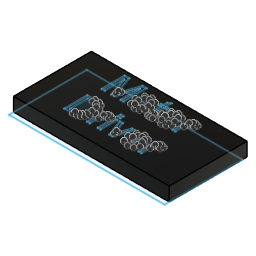
Motor Driver (Autodesk Fusion 360 design; units mm, degrees)
Autodesk Fusion 360 part; units mm, degrees
sketch "sketch 914" plane through (0, 0, 41) normal (0, 0, 1) x (1, 0, 0)
  line L0 (19, -12) -> (-15, -12)
  line L1 (19, 5) -> (19, -12)
  line L2 (-15, 5) -> (19, 5)
  line L3 (-15, -12) -> (-15, 5)
extrude "Extrude1" add sketch "sketch 914" along normal blind 3
sketch "sketch 936" plane through (0, 0, 44) normal (0, 0, 1) x (-1, 0, 0)
  spline S0 degree 3 poles (-7.3462, 7.2033) (-7.4233, 7.1305) (-7.5921, 6.9711) (-7.6781, 6.7547) (-7.7248, 6.6371) knots 0 0 0 0 0.031433 0.068842 0.068842 0.068842 0.068842
  spline S1 degree 3 poles (-6.7698, 7.3806) (-6.8767, 7.3743) (-7.0836, 7.3621) (-7.2607, 7.255) (-7.3462, 7.2033) knots 0 0 0 0 0.031605 0.061119 0.061119 0.061119 0.061119
  spline S2 degree 3 poles (-6.0126, 7.0634) (-6.1207, 7.1559) (-6.339, 7.3427) (-6.6253, 7.3679) (-6.7698, 7.3806) knots 0 0 0 0 0.041584 0.083942 0.083942 0.083942 0.083942
  spline S3 degree 3 poles (-5.675, 6.1494) (-5.6927, 6.3313) (-5.7254, 6.6668) (-5.9224, 6.9388) (-6.0126, 7.0634) knots 0 0 0 0 0.053662 0.09901 0.09901 0.09901 0.09901
  line L0 (-8.3762, 6.1494) -> (-5.675, 6.1494)
  spline S4 degree 3 poles (-8.3796, 5.9857) (-8.3794, 6.0084) (-8.3789, 6.063) (-8.3772, 6.1176) (-8.3762, 6.1494) knots 0 0 0 0 0.006822 0.016375 0.016375 0.016375 0.016375
  spline S5 degree 3 poles (-7.9192, 4.5941) (-8.0532, 4.7859) (-8.3441, 5.202) (-8.3672, 5.7112) (-8.3796, 5.9857) knots 0 0 0 0 0.068809 0.149275 0.149275 0.149275 0.149275
  spline S6 degree 3 poles (-6.7323, 4.0996) (-6.9617, 4.1184) (-7.4113, 4.1554) (-7.7522, 4.4499) (-7.9192, 4.5941) knots 0 0 0 0 0.067144 0.131583 0.131583 0.131583 0.131583
  spline S7 degree 3 poles (-5.5113, 4.6044) (-5.6826, 4.4572) (-6.0337, 4.1556) (-6.4958, 4.1186) (-6.7323, 4.0996) knots 0 0 0 0 0.065997 0.1352 0.1352 0.1352 0.1352
  spline S8 degree 3 poles (-5.0406, 6.0232) (-5.0534, 5.7434) (-5.0771, 5.224) (-5.3742, 4.8) (-5.5113, 4.6044) knots 0 0 0 0 0.082022 0.152248 0.152248 0.152248 0.152248
  spline S9 degree 3 poles (-5.5061, 7.396) (-5.3706, 7.2068) (-5.0776, 6.7982) (-5.0535, 6.294) (-5.0406, 6.0232) knots 0 0 0 0 0.068378 0.147724 0.147724 0.147724 0.147724
  spline S10 degree 3 poles (-6.7664, 7.8854) (-6.5192, 7.869) (-6.0464, 7.8377) (-5.6806, 7.5386) (-5.5061, 7.396) knots 0 0 0 0 0.072283 0.138227 0.138227 0.138227 0.138227
  spline S11 degree 3 poles (-7.8032, 7.5784) (-7.6531, 7.6679) (-7.3343, 7.8578) (-6.9628, 7.8758) (-6.7664, 7.8854) knots 0 0 0 0 0.051631 0.10961 0.10961 0.10961 0.10961
  spline S12 degree 3 poles (-8.3591, 6.7156) (-8.3009, 6.8886) (-8.1881, 7.2236) (-7.9286, 7.4628) (-7.8032, 7.5784) knots 0 0 0 0 0.053808 0.104129 0.104129 0.104129 0.104129
  line L1 (-7.7248, 6.6371) -> (-8.3591, 6.7156)
  spline S13 degree 3 poles (-6.028, 4.8874) (-5.9425, 4.993) (-5.7635, 5.2141) (-5.7277, 5.4969) (-5.7091, 5.6446) knots 0 0 0 0 0.039943 0.083623 0.083623 0.083623 0.083623
  spline S14 degree 3 poles (-6.7391, 4.6044) (-6.6044, 4.6155) (-6.3383, 4.6376) (-6.1305, 4.8049) (-6.028, 4.8874) knots 0 0 0 0 0.039562 0.078122 0.078122 0.078122 0.078122
  spline S15 degree 3 poles (-7.4997, 4.9591) (-7.3943, 4.8556) (-7.1827, 4.6478) (-6.8874, 4.6189) (-6.7391, 4.6044) knots 0 0 0 0 0.042919 0.086214 0.086214 0.086214 0.086214
  spline S16 degree 3 poles (-7.7316, 5.6446) (-7.7161, 5.5075) (-7.6882, 5.2613) (-7.5575, 5.0519) (-7.4997, 4.9591) knots 0 0 0 0 0.040752 0.073178 0.073178 0.073178 0.073178
  line L2 (-5.7091, 5.6446) -> (-7.7316, 5.6446)
  line L3 (-3.3319, 7.8035) -> (-2.7589, 7.8035)
  line L4 (-4.7029, 4.1814) -> (-3.3319, 7.8035)
  line L5 (-4.072, 4.1814) -> (-4.7029, 4.1814)
  line L6 (-3.2671, 6.3915) -> (-4.072, 4.1814)
  spline S17 degree 3 poles (-3.0385, 7.0805) (-3.0704, 6.9751) (-3.1404, 6.7434) (-3.2224, 6.5156) (-3.2671, 6.3915) knots 0 0 0 0 0.033037 0.072597 0.072597 0.072597 0.072597
  spline S18 degree 3 poles (-2.8066, 6.3506) (-2.848, 6.4696) (-2.932, 6.7108) (-3.0027, 6.9562) (-3.0385, 7.0805) knots 0 0 0 0 0.037803 0.076597 0.076597 0.076597 0.076597
  line L7 (-2.029, 4.1814) -> (-2.8066, 6.3506)
  line L8 (-1.381, 4.1814) -> (-2.029, 4.1814)
  line L9 (-2.7589, 7.8035) -> (-1.381, 4.1814)
  line L10 (-0.8182, 7.8035) -> (-0.2043, 7.8035)
  line L11 (-0.8182, 4.1814) -> (-0.8182, 7.8035)
  line L12 (-0.2043, 4.1814) -> (-0.8182, 4.1814)
  line L13 (-0.2043, 7.8035) -> (-0.2043, 4.1814)
  line L14 (-0.8182, 3.5095) -> (-0.2043, 3.5095)
  line L15 (-0.8182, 2.8035) -> (-0.8182, 3.5095)
  line L16 (-0.2043, 2.8035) -> (-0.8182, 2.8035)
  line L17 (-0.2043, 3.5095) -> (-0.2043, 2.8035)
  line L18 (1.5181, 7.8035) -> (2.132, 7.8035)
  line L19 (1.5181, 5.9072) -> (1.5181, 7.8035)
  spline S19 degree 3 poles (1.4158, 5.191) (1.4456, 5.3046) (1.5072, 5.5394) (1.5144, 5.782) (1.5181, 5.9072) knots 0 0 0 0 0.035125 0.072559 0.072559 0.072559 0.072559
  spline S20 degree 3 poles (1.1872, 4.855) (1.2372, 4.9004) (1.3402, 4.9939) (1.3901, 5.124) (1.4158, 5.191) knots 0 0 0 0 0.019933 0.041138 0.041138 0.041138 0.041138
  spline S21 degree 3 poles (0.8257, 4.734) (0.8911, 4.739) (1.0217, 4.7491) (1.1321, 4.8197) (1.1872, 4.855) knots 0 0 0 0 0.019338 0.038658 0.038658 0.038658 0.038658
  spline S22 degree 3 poles (0.3755, 4.867) (0.4489, 4.8282) (0.5902, 4.7536) (0.7493, 4.7403) (0.8257, 4.734) knots 0 0 0 0 0.024622 0.047376 0.047376 0.047376 0.047376
  line L20 (0.1641, 4.2974) -> (0.3755, 4.867)
  spline S23 degree 3 poles (0.795, 4.0996) (0.6887, 4.1094) (0.4645, 4.1301) (0.2676, 4.2398) (0.1641, 4.2974) knots 0 0 0 0 0.031681 0.066776 0.066776 0.066776 0.066776
  spline S24 degree 3 poles (1.189, 4.2224) (1.1279, 4.1866) (1.0061, 4.1151) (0.8652, 4.1048) (0.795, 4.0996) knots 0 0 0 0 0.020935 0.041755 0.041755 0.041755 0.041755
  spline S25 degree 3 poles (1.5795, 4.7306) (1.5179, 4.619) (1.4132, 4.4292) (1.2544, 4.2827) (1.189, 4.2224) knots 0 0 0 0 0.037894 0.064453 0.064453 0.064453 0.064453
  line L21 (1.5795, 4.1814) -> (1.5795, 4.7306)
  line L22 (2.132, 4.1814) -> (1.5795, 4.1814)
  line L23 (2.132, 7.8035) -> (2.132, 4.1814)
  line L24 (-9.737, 7.8035) -> (-9.1231, 7.8035)
  line L25 (-9.737, 5.9072) -> (-9.737, 7.8035)
  spline S26 degree 3 poles (-9.8394, 5.191) (-9.8095, 5.3046) (-9.7479, 5.5394) (-9.7407, 5.782) (-9.737, 5.9072) knots 0 0 0 0 0.035125 0.072559 0.072559 0.072559 0.072559
  spline S27 degree 3 poles (-10.0679, 4.855) (-10.018, 4.9004) (-9.9149, 4.9939) (-9.8651, 5.124) (-9.8394, 5.191) knots 0 0 0 0 0.019933 0.041138 0.041138 0.041138 0.041138
  spline S28 degree 3 poles (-10.4294, 4.734) (-10.364, 4.739) (-10.2334, 4.7491) (-10.123, 4.8197) (-10.0679, 4.855) knots 0 0 0 0 0.019338 0.038658 0.038658 0.038658 0.038658
  spline S29 degree 3 poles (-10.8796, 4.867) (-10.8062, 4.8282) (-10.6649, 4.7536) (-10.5058, 4.7403) (-10.4294, 4.734) knots 0 0 0 0 0.024622 0.047376 0.047376 0.047376 0.047376
  line L26 (-11.0911, 4.2974) -> (-10.8796, 4.867)
  spline S30 degree 3 poles (-10.4601, 4.0996) (-10.5664, 4.1094) (-10.7906, 4.1301) (-10.9876, 4.2398) (-11.0911, 4.2974) knots 0 0 0 0 0.031681 0.066775 0.066775 0.066775 0.066775
  spline S31 degree 3 poles (-10.0662, 4.2224) (-10.1272, 4.1866) (-10.2491, 4.1151) (-10.3899, 4.1048) (-10.4601, 4.0996) knots 0 0 0 0 0.020935 0.041755 0.041755 0.041755 0.041755
  spline S32 degree 3 poles (-9.6756, 4.7306) (-9.7372, 4.619) (-9.8419, 4.4292) (-10.0007, 4.2827) (-10.0662, 4.2224) knots 0 0 0 0 0.037894 0.064453 0.064453 0.064453 0.064453
  line L27 (-9.6756, 4.1814) -> (-9.6756, 4.7306)
  line L28 (-9.1231, 4.1814) -> (-9.6756, 4.1814)
  line L29 (-9.1231, 7.8035) -> (-9.1231, 4.1814)
  line L30 (5.2868, 7.8035) -> (7.0911, 7.8035)
  spline S33 degree 3 poles (4.4836, 7.7183) (4.6084, 7.7431) (4.8735, 7.7959) (5.1438, 7.8009) (5.2868, 7.8035) knots 0 0 0 0 0.0381 0.080914 0.080914 0.080914 0.080914
  spline S34 degree 3 poles (3.8868, 7.4676) (3.976, 7.52) (4.1637, 7.6302) (4.3736, 7.688) (4.4836, 7.7183) knots 0 0 0 0 0.030916 0.064986 0.064986 0.064986 0.064986
  spline S35 degree 3 poles (3.4314, 7.014) (3.5004, 7.1035) (3.6323, 7.2749) (3.8045, 7.4053) (3.8868, 7.4676) knots 0 0 0 0 0.03373 0.064527 0.064527 0.064527 0.064527
  spline S36 degree 3 poles (3.0904, 6.2858) (3.1353, 6.4225) (3.2196, 6.6792) (3.364, 6.9073) (3.4314, 7.014) knots 0 0 0 0 0.042972 0.080682 0.080682 0.080682 0.080682
  spline S37 degree 3 poles (2.9574, 5.2763) (2.9616, 5.4563) (2.9696, 5.7977) (3.0516, 6.1291) (3.0904, 6.2858) knots 0 0 0 0 0.05382 0.1021 0.1021 0.1021 0.1021
  spline S38 degree 3 poles (3.1535, 4.0877) (3.0963, 4.272) (2.9763, 4.659) (2.9639, 5.0641) (2.9574, 5.2763) knots 0 0 0 0 0.05763 0.12096 0.12096 0.12096 0.12096
  spline S39 degree 3 poles (3.7452, 3.2333) (3.6211, 3.354) (3.3681, 3.6) (3.2259, 3.9231) (3.1535, 4.0877) knots 0 0 0 0 0.051428 0.1048 0.1048 0.1048 0.1048
  spline S40 degree 3 poles (4.4785, 2.8752) (4.3419, 2.9136) (4.0756, 2.9886) (3.8534, 3.1532) (3.7452, 3.2333) knots 0 0 0 0 0.042175 0.082214 0.082214 0.082214 0.082214
  spline S41 degree 3 poles (5.3687, 2.8035) (5.1968, 2.8043) (4.8981, 2.8055) (4.6036, 2.8544) (4.4785, 2.8752) knots 0 0 0 0 0.051447 0.089431 0.089431 0.089431 0.089431
  line L31 (7.0911, 2.8035) -> (5.3687, 2.8035)
  line L32 (7.0911, 7.8035) -> (7.0911, 2.8035)
  line L33 (6.4294, 3.3936) -> (6.4294, 7.2135)
  line L34 (5.3789, 3.3936) -> (6.4294, 3.3936)
  spline S42 degree 3 poles (4.5229, 3.4959) (4.638, 3.4663) (4.9182, 3.3942) (5.2081, 3.3938) (5.3789, 3.3936) knots 0 0 0 0 0.035542 0.08651 0.08651 0.08651 0.08651
  spline S43 degree 3 poles (3.897, 4.0604) (3.9833, 3.9332) (4.1463, 3.6934) (4.4024, 3.559) (4.5229, 3.4959) knots 0 0 0 0 0.045283 0.085444 0.085444 0.085444 0.085444
  spline S44 degree 3 poles (3.6395, 5.266) (3.644, 5.0309) (3.6521, 4.6111) (3.8222, 4.2286) (3.897, 4.0604) knots 0 0 0 0 0.069662 0.124385 0.124385 0.124385 0.124385
  spline S45 degree 3 poles (3.7708, 6.2295) (3.7326, 6.0838) (3.6498, 5.7682) (3.6431, 5.4417) (3.6395, 5.266) knots 0 0 0 0 0.045044 0.097543 0.097543 0.097543 0.097543
  spline S46 degree 3 poles (4.1374, 6.8622) (4.0622, 6.7735) (3.9022, 6.5848) (3.8163, 6.3526) (3.7708, 6.2295) knots 0 0 0 0 0.034627 0.073625 0.073625 0.073625 0.073625
  spline S47 degree 3 poles (4.5859, 7.1214) (4.4988, 7.0894) (4.3341, 7.0289) (4.2004, 6.9156) (4.1374, 6.8622) knots 0 0 0 0 0.027605 0.052162 0.052162 0.052162 0.052162
  spline S48 degree 3 poles (5.3619, 7.2135) (5.214, 7.2121) (4.9517, 7.2095) (4.697, 7.1482) (4.5859, 7.1214) knots 0 0 0 0 0.044185 0.078357 0.078357 0.078357 0.078357
  line L35 (6.4294, 7.2135) -> (5.3619, 7.2135)
  line L36 (-9.3516, 0) -> (-8.7377, 0)
  line L37 (-9.3516, -1.8963) -> (-9.3516, 0)
  spline S49 degree 3 poles (-9.454, -2.6126) (-9.4241, -2.4989) (-9.3625, -2.2642) (-9.3553, -2.0215) (-9.3516, -1.8963) knots 0 0 0 0 0.035125 0.07256 0.07256 0.07256 0.07256
  spline S50 degree 3 poles (-9.6825, -2.9485) (-9.6325, -2.9032) (-9.5295, -2.8097) (-9.4797, -2.6796) (-9.454, -2.6126) knots 0 0 0 0 0.019933 0.041138 0.041138 0.041138 0.041138
  spline S51 degree 3 poles (-10.044, -3.0696) (-9.9786, -3.0645) (-9.848, -3.0545) (-9.7376, -2.9838) (-9.6825, -2.9485) knots 0 0 0 0 0.019338 0.038658 0.038658 0.038658 0.038658
  spline S52 degree 3 poles (-10.4942, -2.9366) (-10.4208, -2.9753) (-10.2795, -3.05) (-10.1204, -3.0632) (-10.044, -3.0696) knots 0 0 0 0 0.024622 0.047376 0.047376 0.047376 0.047376
  line L38 (-10.7057, -3.5061) -> (-10.4942, -2.9366)
  spline S53 degree 3 poles (-10.0747, -3.704) (-10.181, -3.6942) (-10.4052, -3.6735) (-10.6022, -3.5638) (-10.7057, -3.5061) knots 0 0 0 0 0.031681 0.066775 0.066775 0.066775 0.066775
  spline S54 degree 3 poles (-9.6808, -3.5812) (-9.7418, -3.617) (-9.8637, -3.6884) (-10.0045, -3.6988) (-10.0747, -3.704) knots 0 0 0 0 0.020935 0.041755 0.041755 0.041755 0.041755
  spline S55 degree 3 poles (-9.2902, -3.073) (-9.3518, -3.1846) (-9.4565, -3.3743) (-9.6153, -3.5208) (-9.6808, -3.5812) knots 0 0 0 0 0.037894 0.064453 0.064453 0.064453 0.064453
  line L39 (-9.2902, -3.6221) -> (-9.2902, -3.073)
  line L40 (-8.7377, -3.6221) -> (-9.2902, -3.6221)
  line L41 (-8.7377, 0) -> (-8.7377, -3.6221)
  spline S56 degree 3 poles (-5.1003, -0.4059) (-4.9637, -0.5975) (-4.6656, -1.0159) (-4.6434, -1.5315) (-4.6313, -1.8111) knots 0 0 0 0 0.069132 0.150979 0.150979 0.150979 0.150979
  spline S57 degree 3 poles (-6.3298, 0.0819) (-6.0912, 0.0644) (-5.6293, 0.0305) (-5.2727, -0.2637) (-5.1003, -0.4059) knots 0 0 0 0 0.06984 0.135217 0.135217 0.135217 0.135217
  spline S58 degree 3 poles (-7.2046, -0.1398) (-7.0673, -0.0752) (-6.7901, 0.0553) (-6.4842, 0.073) (-6.3298, 0.0819) knots 0 0 0 0 0.045086 0.090997 0.090997 0.090997 0.090997
  spline S59 degree 3 poles (-7.8151, -0.7623) (-7.737, -0.636) (-7.5803, -0.3827) (-7.3301, -0.221) (-7.2046, -0.1398) knots 0 0 0 0 0.043936 0.088163 0.088163 0.088163 0.088163
  spline S60 degree 3 poles (-8.0249, -1.8622) (-8.0208, -1.6513) (-8.0134, -1.2718) (-7.8761, -0.919) (-7.8151, -0.7623) knots 0 0 0 0 0.062677 0.112748 0.112748 0.112748 0.112748
  spline S61 degree 3 poles (-7.5508, -3.2145) (-7.6889, -3.0274) (-7.9846, -2.6269) (-8.0109, -2.128) (-8.0249, -1.8622) knots 0 0 0 0 0.068269 0.146129 0.146129 0.146129 0.146129
  spline S62 degree 3 poles (-6.3298, -3.704) (-6.5652, -3.6858) (-7.0242, -3.6503) (-7.3783, -3.3573) (-7.5508, -3.2145) knots 0 0 0 0 0.068966 0.13445 0.13445 0.13445 0.13445
  spline S63 degree 3 poles (-5.1907, -3.3015) (-5.3575, -3.4189) (-5.6991, -3.6593) (-6.1163, -3.6888) (-6.3298, -3.704) knots 0 0 0 0 0.059989 0.122873 0.122873 0.122873 0.122873
  spline S64 degree 3 poles (-4.6313, -1.8111) (-4.6453, -2.1159) (-4.671, -2.6767) (-5.0278, -3.1057) (-5.1907, -3.3015) knots 0 0 0 0 0.088678 0.163104 0.163104 0.163104 0.163104
  spline S65 degree 3 poles (-5.5658, -2.8513) (-5.4776, -2.7111) (-5.2787, -2.395) (-5.2681, -2.0198) (-5.2623, -1.8111) knots 0 0 0 0 0.048858 0.110125 0.110125 0.110125 0.110125
  spline S66 degree 3 poles (-6.3298, -3.1958) (-6.1829, -3.1815) (-5.8893, -3.1529) (-5.6736, -2.9518) (-5.5658, -2.8513) knots 0 0 0 0 0.042993 0.085916 0.085916 0.085916 0.085916
  spline S67 degree 3 poles (-7.0887, -2.8496) (-6.9811, -2.9506) (-6.7671, -3.1515) (-6.4751, -3.1811) (-6.3298, -3.1958) knots 0 0 0 0 0.042966 0.085508 0.085508 0.085508 0.085508
  spline S68 degree 3 poles (-7.3939, -1.8315) (-7.3873, -2.0344) (-7.3752, -2.4025) (-7.1775, -2.7111) (-7.0887, -2.8496) knots 0 0 0 0 0.059538 0.108042 0.108042 0.108042 0.108042
  spline S69 degree 3 poles (-7.0904, -0.7708) (-7.1786, -0.9134) (-7.3785, -1.2364) (-7.3884, -1.6182) (-7.3939, -1.8315) knots 0 0 0 0 0.049463 0.112083 0.112083 0.112083 0.112083
  spline S70 degree 3 poles (-6.3298, -0.4229) (-6.4759, -0.4376) (-6.7689, -0.467) (-6.983, -0.6693) (-7.0904, -0.7708) knots 0 0 0 0 0.042759 0.085769 0.085769 0.085769 0.085769
  spline S71 degree 3 poles (-5.5658, -0.7691) (-5.6735, -0.6681) (-5.889, -0.4662) (-6.1829, -0.4373) (-6.3298, -0.4229) knots 0 0 0 0 0.043 0.086001 0.086001 0.086001 0.086001
  spline S72 degree 3 poles (-5.2623, -1.8111) (-5.2682, -1.6022) (-5.2788, -1.2265) (-5.4776, -0.9097) (-5.5658, -0.7691) knots 0 0 0 0 0.061309 0.11028 0.11028 0.11028 0.11028
  spline S73 degree 3 poles (-3.9901, -0.5252) (-4.0297, -0.5266) (-4.1199, -0.5298) (-4.2093, -0.5422) (-4.2595, -0.5491) knots 0 0 0 0 0.011867 0.027065 0.027065 0.027065 0.027065
  spline S74 degree 3 poles (-3.7804, -0.5696) (-3.8096, -0.5567) (-3.8762, -0.5274) (-3.9492, -0.526) (-3.9901, -0.5252) knots 0 0 0 0 0.00951 0.021627 0.021627 0.021627 0.021627
  spline S75 degree 3 poles (-3.6746, -0.6889) (-3.6873, -0.6651) (-3.7129, -0.6169) (-3.7577, -0.5855) (-3.7804, -0.5696) knots 0 0 0 0 0.007972 0.016149 0.016149 0.016149 0.016149
  spline S76 degree 3 poles (-3.6422, -1.0266) (-3.6413, -0.9543) (-3.6399, -0.8403) (-3.6653, -0.7295) (-3.6746, -0.6889) knots 0 0 0 0 0.021587 0.03402 0.03402 0.03402 0.03402
  line L42 (-3.6422, -3.1446) -> (-3.6422, -1.0266)
  line L43 (-4.2595, -3.1446) -> (-3.6422, -3.1446)
  line L44 (-4.2595, -3.6221) -> (-4.2595, -3.1446)
  line L45 (-3.6422, -3.6221) -> (-4.2595, -3.6221)
  line L46 (-3.6422, -4.8874) -> (-3.6422, -3.6221)
  line L47 (-3.0317, -4.5191) -> (-3.6422, -4.8874)
  line L48 (-3.0317, -3.6221) -> (-3.0317, -4.5191)
  line L49 (-2.5815, -3.6221) -> (-3.0317, -3.6221)
  line L50 (-2.5815, -3.1446) -> (-2.5815, -3.6221)
  line L51 (-3.0317, -3.1446) -> (-2.5815, -3.1446)
  line L52 (-3.0317, -1.0607) -> (-3.0317, -3.1446)
  spline S77 degree 3 poles (-3.1068, -0.3359) (-3.0852, -0.4247) (-3.0275, -0.6622) (-3.0301, -0.9072) (-3.0317, -1.0607) knots 0 0 0 0 0.027317 0.073101 0.073101 0.073101 0.073101
  spline S78 degree 3 poles (-3.366, -0.058) (-3.3096, -0.095) (-3.2004, -0.1666) (-3.1373, -0.2808) (-3.1068, -0.3359) knots 0 0 0 0 0.019896 0.03852 0.03852 0.03852 0.03852
  spline S79 degree 3 poles (-3.8844, 0.0477) (-3.784, 0.0458) (-3.6042, 0.0424) (-3.4389, -0.0273) (-3.366, -0.058) knots 0 0 0 0 0.02979 0.053335 0.053335 0.053335 0.053335
  spline S80 degree 3 poles (-4.3482, -0.0068) (-4.2666, 0.0091) (-4.1133, 0.0389) (-3.9573, 0.0449) (-3.8844, 0.0477) knots 0 0 0 0 0.024895 0.046766 0.046766 0.046766 0.046766
  line L53 (-4.2595, -0.5491) -> (-4.3482, -0.0068)
  spline S81 degree 3 poles (0.7251, -0.4059) (0.8616, -0.5975) (1.1598, -1.0159) (1.182, -1.5315) (1.1941, -1.8111) knots 0 0 0 0 0.069132 0.150979 0.150979 0.150979 0.150979
  spline S82 degree 3 poles (-0.5044, 0.0819) (-0.2658, 0.0644) (0.1961, 0.0305) (0.5527, -0.2637) (0.7251, -0.4059) knots 0 0 0 0 0.06984 0.135217 0.135217 0.135217 0.135217
  spline S83 degree 3 poles (-1.3793, -0.1398) (-1.2419, -0.0752) (-0.9647, 0.0553) (-0.6588, 0.073) (-0.5044, 0.0819) knots 0 0 0 0 0.045086 0.090997 0.090997 0.090997 0.090997
  spline S84 degree 3 poles (-1.9898, -0.7623) (-1.9117, -0.636) (-1.755, -0.3827) (-1.5048, -0.221) (-1.3793, -0.1398) knots 0 0 0 0 0.043936 0.088163 0.088163 0.088163 0.088163
  spline S85 degree 3 poles (-2.1995, -1.8622) (-2.1954, -1.6513) (-2.1881, -1.2718) (-2.0508, -0.919) (-1.9898, -0.7623) knots 0 0 0 0 0.062677 0.112748 0.112748 0.112748 0.112748
  spline S86 degree 3 poles (-1.7254, -3.2145) (-1.8636, -3.0274) (-2.1592, -2.6269) (-2.1855, -2.128) (-2.1995, -1.8622) knots 0 0 0 0 0.068269 0.146129 0.146129 0.146129 0.146129
  spline S87 degree 3 poles (-0.5044, -3.704) (-0.7399, -3.6858) (-1.1989, -3.6503) (-1.553, -3.3573) (-1.7254, -3.2145) knots 0 0 0 0 0.068966 0.13445 0.13445 0.13445 0.13445
  spline S88 degree 3 poles (0.6347, -3.3015) (0.4679, -3.4189) (0.1263, -3.6593) (-0.2909, -3.6888) (-0.5044, -3.704) knots 0 0 0 0 0.059989 0.122873 0.122873 0.122873 0.122873
  spline S89 degree 3 poles (1.1941, -1.8111) (1.1801, -2.1159) (1.1543, -2.6767) (0.7975, -3.1057) (0.6347, -3.3015) knots 0 0 0 0 0.088678 0.163104 0.163104 0.163104 0.163104
  spline S90 degree 3 poles (0.2596, -2.8513) (0.3478, -2.7111) (0.5467, -2.395) (0.5572, -2.0198) (0.5631, -1.8111) knots 0 0 0 0 0.048858 0.110125 0.110125 0.110125 0.110125
  spline S91 degree 3 poles (-0.5044, -3.1958) (-0.3575, -3.1815) (-0.064, -3.1529) (0.1518, -2.9518) (0.2596, -2.8513) knots 0 0 0 0 0.042993 0.085916 0.085916 0.085916 0.085916
  spline S92 degree 3 poles (-1.2633, -2.8496) (-1.1557, -2.9506) (-0.9417, -3.1515) (-0.6497, -3.1811) (-0.5044, -3.1958) knots 0 0 0 0 0.042966 0.085508 0.085508 0.085508 0.085508
  spline S93 degree 3 poles (-1.5686, -1.8315) (-1.5619, -2.0344) (-1.5499, -2.4025) (-1.3521, -2.7111) (-1.2633, -2.8496) knots 0 0 0 0 0.059538 0.108042 0.108042 0.108042 0.108042
  spline S94 degree 3 poles (-1.265, -0.7708) (-1.3532, -0.9134) (-1.5531, -1.2364) (-1.563, -1.6182) (-1.5686, -1.8315) knots 0 0 0 0 0.049463 0.112083 0.112083 0.112083 0.112083
  spline S95 degree 3 poles (-0.5044, -0.4229) (-0.6505, -0.4376) (-0.9436, -0.467) (-1.1577, -0.6693) (-1.265, -0.7708) knots 0 0 0 0 0.04276 0.085769 0.085769 0.085769 0.085769
  spline S96 degree 3 poles (0.2596, -0.7691) (0.1518, -0.6681) (-0.0636, -0.4662) (-0.3575, -0.4373) (-0.5044, -0.4229) knots 0 0 0 0 0.043 0.086001 0.086001 0.086001 0.086001
  spline S97 degree 3 poles (0.5631, -1.8111) (0.5572, -1.6022) (0.5465, -1.2265) (0.3478, -0.9097) (0.2596, -0.7691) knots 0 0 0 0 0.061309 0.11028 0.11028 0.11028 0.11028
  line L54 (6.0883, 0) -> (6.7261, 0)
  line L55 (6.0883, -4.2565) -> (6.0883, 0)
  line L56 (4.6422, 0) -> (6.0883, -4.2565)
  line L57 (4.0454, 0) -> (4.6422, 0)
  line L58 (2.5924, -4.1849) -> (4.0454, 0)
  line L59 (2.5924, 0) -> (2.5924, -4.1849)
  line L60 (1.9546, 0) -> (2.5924, 0)
  line L61 (1.9546, -5) -> (1.9546, 0)
  line L62 (2.8448, -5) -> (1.9546, -5)
  line L63 (4.042, -1.5211) -> (2.8448, -5)
  spline S98 degree 3 poles (4.308, -0.7196) (4.2719, -0.832) (4.1858, -1.1) (4.0948, -1.3664) (4.042, -1.5211) knots 0 0 0 0 0.035404 0.084451 0.084451 0.084451 0.084451
  spline S99 degree 3 poles (4.5467, -1.4598) (4.4991, -1.3158) (4.4177, -1.0697) (4.3402, -0.8223) (4.308, -0.7196) knots 0 0 0 0 0.045488 0.077767 0.077767 0.077767 0.077767
  line L64 (5.7302, -5) -> (4.5467, -1.4598)
  line L65 (6.7261, -5) -> (5.7302, -5)
  line L66 (6.7261, 0) -> (6.7261, -5)
extrude "Extrude2" cut sketch "sketch 936" against normal blind 0.5
extrude "Extrude3" cut 1 faces at (7.6667, -12, 42) along direction (0, 1, 0) blind 1
extrude "Extrude4" add 1 faces at (12.0151, 5, 42.8333) along direction (0, 1, 0) blind 1
extrude "Extrude5" add 1 faces at (-5.7302, 5.3333, 43.8333) along direction (-1, 0, 0) mid plane 11
